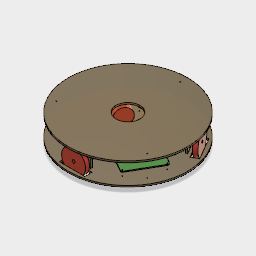
prototype (Autodesk Fusion 360 design; units mm, degrees)
Autodesk Fusion 360 part; units mm, degrees
note: some values were not read from the file. Chosen so that the rebuilt part matches the saved one: which face or edge a step refers to. Set by a fixed rule: which sketch regions a step uses.
cylinder "CylinderPrimitive1" add diameter 33 height 29 placed x (1, 0, 0) y (0, 1, 0) z (0, 0, 1) at (0, 0, 0) makes body 1 in component "motor"
cylinder "CylinderPrimitive2" add diameter 37 height 24 placed x (1, 0, 0) y (0, 1, 0) z (0, 0, 1) at (0, 0, 29) bodies 1 in component "motor"
sketch "Sketch3" plane through (0, 0, 53) normal (0, 0, 1) x (1, 0, 0) in component "motor"
  circle A0 centre (0, 0) radius 18.5
  line L0 (0, 0) -> (0, 7)
  circle A1 centre (0, 7) radius 6
  circle A2 centre (0, 0) radius 15.5
  circle A3 centre (-15.5, 0) radius 1.5
  circle A4 centre (-7.75, -13.4234) radius 1.5
  circle A5 centre (7.75, -13.4234) radius 1.5
  circle A6 centre (15.5, 0) radius 1.5
  circle A7 centre (7.75, 13.4234) radius 1.5
  circle A8 centre (-7.75, 13.4234) radius 1.5
  dimension "d7" = 7
  dimension "d8" = 12
  dimension "d13" = 31
  dimension "d14" = 3
  dimension "d20" = 360
  measures "d7" distance of A0.centre L0.end
  measures "d8" diameter of A1
  measures "d13" diameter of A2
  measures "d14" diameter of A3
cylinder "CylinderPrimitive3" add diameter 12 height 6 placed x (1, 0, 0) y (0, 1, 0) z (0, 0, 1) at (0, 7, 53) bodies 1 in component "motor"
cylinder "CylinderPrimitive4" add diameter 6 height 21 placed x (1, 0, 0) y (0, 1, 0) z (0, 0, 1) at (0, 7, 53) bodies 1 in component "motor"
extrude "Extrude2" cut sketch "Sketch3" against normal blind 10 contours A2 A6 | A2 A6 | A2 A7 | A2 A7 | A2 A5 | A2 A5 | A2 A8 | A2 A8 | A2 A4 | A2 A4 | A2 A3 | A2 A3 bodies 1 in component "motor"
move_face "OffsetFaces1" offset 15 1 faces at (4.8173, 3.9832, 0) on bodies 1 in component "motor"
sketch "Sketch7" plane through (0, 0, 29) normal (0, 0, -1) x (-1, 0, 0) in component "motor"
  circle A0 centre (0, 0) radius 18.5
  circle A1 centre (0, 0) radius 16.5
sketch "Sketch6" plane through (0, 0, 0) normal (0, 1, 0) x (1, 0, 0)
  line L0 (306.1493, 283.3069) -> (269.5493, 283.3069)
  line L1 (266.3493, 280.1069) -> (266.3493, 211.5069)
  line L2 (309.3493, 211.5069) -> (309.3493, 280.1069)
  line L3 (306.1493, 208.3069) -> (306.1493, 208.3069)
  arc A0 (306.1493, 208.3069) -> (309.3493, 211.5069) centre (306.1493, 211.5069) ccw
  arc A1 (266.3493, 211.5069) -> (269.5493, 208.3069) centre (269.5493, 211.5069) ccw
  arc A2 (309.3493, 280.1069) -> (306.1493, 283.3069) centre (306.1493, 280.1069) ccw
  arc A3 (269.5493, 283.3069) -> (266.3493, 280.1069) centre (269.5493, 280.1069) ccw
  line L4 (306.1493, 208.3069) -> (269.5493, 208.3069)
  line L5 (155.099, 257.3507) -> (209.099, 257.3507)
  line L6 (209.099, 257.3507) -> (209.099, 155.3507)
  line L7 (209.099, 155.3507) -> (155.099, 155.3507)
  line L8 (155.099, 155.3507) -> (155.099, 257.3507)
  circle A4 centre (269.5493, 211.5069) radius 1
  circle A5 centre (306.1493, 211.5069) radius 1
  circle A6 centre (269.5493, 280.1069) radius 1
  circle A7 centre (306.1493, 280.1069) radius 1
  dimension "d71" = 3.2
  dimension "d72" = 3.2
  dimension "d74" = 3.2
  dimension "d81" = 54
  dimension "d82" = 102
  dimension "d132" = 2
  dimension "d133" = 2
  dimension "d134" = 2
  dimension "d135" = 2
  measures "d71" radius of A0
  measures "d72" radius of A1
  measures "d74" radius of A3
  measures "d81" distance of L5.start L5.end
  measures "d82" distance of L5.start L7.end
  measures "d132" diameter of A4
  measures "d133" diameter of A5
  measures "d134" diameter of A6
  measures "d135" diameter of A7
move_body "Move6" bodies 1 to x (-1, 0, 0) y (0, -1, 0) z (0, 0, 1) at (0, 0, 0) in component "motor"
cylinder "CylinderPrimitive5" add diameter 60 height -11 placed x (1, 0, 0) y (0, 1, 0) z (0, 0, 1) at (0, -7, 74) separate body makes body 2 in component "motor"
sketch "Sketch10" plane through (0, 0, 0) normal (1, 0, 0) x (0, 0, -1)
  line L0 (40, 0) -> (40, 40)
other "C-Pattern5"
cylinder "CylinderPrimitive6" add diameter 50 height -8.5 placed x (1, 0, 0) y (0, 1, 0) z (0, 0, 1) at (0, -7, 74) separate body makes body 3 in component "motor"
move_body "Move7" bodies 2 to x (1, 0, 0) y (0, 1, 0) z (0, 0, 1) at (0, 0, 2) in component "motor"
move_face "OffsetFaces2" offset 2 1 faces at (7.6631, 4.2397, 65) on bodies 2 in component "motor"
sketch "Sketch12" plane through (0, -22.6, 0) normal (0, 1, 0) x (-1, 0, 0)
  line L0 (25.625, 76) -> (25.625, 63)
  line L1 (25.625, 63) -> (-25.625, 63)
  line L2 (-25.625, 63) -> (-25.625, 76)
  line L3 (-25.625, 76) -> (25.625, 76)
  circle A0 centre (0, -40) radius 125
  line L4 (25.625, 63) -> (-25.625, 63)
  line L5 (-25.625, 63) -> (-25.625, 76)
  line L6 (-25.625, 76) -> (25.625, 76)
  line L7 (25.625, 76) -> (25.625, 63)
  line L8 (-26.625, 77) -> (26.625, 77)
  line L9 (26.625, 77) -> (26.625, 62)
  line L10 (26.625, 62) -> (-26.625, 62)
  line L11 (-26.625, 62) -> (-26.625, 77)
  line L12 (-88.0125, -121.5579) -> (-114.6375, -75.4421)
  line L13 (-114.6375, -75.4421) -> (-101.6471, -67.9421)
  line L14 (-101.6471, -67.9421) -> (-75.0221, -114.0579)
  line L15 (-75.0221, -114.0579) -> (-88.0125, -121.5579)
  line L16 (114.6375, -75.4421) -> (88.0125, -121.5579)
  line L17 (88.0125, -121.5579) -> (75.0221, -114.0579)
  line L18 (75.0221, -114.0579) -> (101.6471, -67.9421)
  line L19 (101.6471, -67.9421) -> (114.6375, -75.4421)
  dimension "d127" = 1
  dimension "d129" = 360
extrude "Extrude1" add sketch "Sketch12" along normal blind 3.4 separate body contours A0 makes body 4 in component "base"
extrude "Extrude1'" add sketch "Sketch6" along normal blind 2 separate body contours L0 L1 L2 A0 A1 A2 A3 L4 makes body 5 in component "motordriver"
move_body "Move1" bodies 5 to x (0, 0, 1) y (0, 1, 0) z (-1, 0, 0) at (-246.0336, 0, -405.0116) in component "motordriver"
sketch "Sketch13" plane through (0, 0, 53) normal (0, 0, 1) x (1, 0, 0)
  line L0 (125, -19.2) -> (-125, -19.2)
  line L1 (0, 24) -> (0, -19.2) construction
  line L2 (125, -22.6) -> (-125, -22.6)
  circle A0 centre (-7.75, 13.4234) radius 1
  circle A1 centre (0, 0) radius 16.5
  circle A2 centre (0, 0) radius 16.5
  circle A3 centre (7.75, 13.4234) radius 1
  circle A4 centre (15.5, 0) radius 1
  circle A5 centre (7.75, -13.4234) radius 1
  circle A6 centre (-7.75, -13.4234) radius 1
  circle A7 centre (-15.5, 0) radius 1
  circle A8 centre (0, 0) radius 18.5
  line L3 (-18.5, 0) -> (-18.5, -22.6)
  line L4 (18.4998, 0.0775) -> (18.5948, -22.6)
  arc A9 (18.4998, 0.0775) -> (-18.5, 0) centre (0, 0) ccw
  line L5 (-18.5, -22.6) -> (18.5948, -22.6)
  circle A10 centre (0, -7) radius 6.5
  point P0 (-7.75, 13.4234)
  point P1 (7.75, 13.4234)
  point P2 (15.5, 0)
  point P3 (16.5, 0)
  point P4 (7.75, -13.4234)
  point P5 (-7.75, -13.4234)
  point P6 (-15.5, 0)
  dimension "d140" = 13
  measures "d140" diameter of A10
extrude "Extrude1''" add sketch "Sketch13" along normal blind 3.4 separate body contours L0 L2 L3 L4 L5 | L0 A8 L3 L4 | A8 L4 A9 | A1 A2 makes body 6 in component "motorHolder"
other "C-Pattern6"
combine "Combine1" operation cut target body 4 tool bodies 6 body 6 seen with x (-0.5, 0, -0.866025) y (0, 1, 0) z (0.866025, 0, -0.5) at (34.641, 0, -60) keep tools in component "base"
combine "Combine2" operation cut target body 4 tool bodies 6 keep tools in component "base"
combine "Combine3" operation cut target body 4 tool bodies 6 body 6 seen with x (-0.5, 0, 0.866025) y (0, 1, 0) z (-0.866025, 0, -0.5) at (-34.641, 0, -60) keep tools in component "base"
other "C-Pattern7"
sketch "Sketch14" plane through (0, -8, 0) normal (0, 1, 0) x (-1, 0, 0)
  circle A0 centre (-33.9396, 18.9394) radius 1
  circle A1 centre (-99.9361, -22.1699) radius 1
  circle A2 centre (-68.2396, -40.4699) radius 1
  circle A3 centre (-65.6361, 37.2394) radius 1
  line L0 (0, -40) -> (-1.5, -40)
  circle A4 centre (34.5267, -135.4623) radius 1
  circle A5 centre (-34.0733, -98.8623) radius 1
  circle A6 centre (-34.0733, -135.4623) radius 1
  circle A7 centre (34.5267, -98.8623) radius 1
  circle A8 centre (65.4094, 37.6322) radius 1
  circle A9 centre (68.0129, -40.0772) radius 1
  circle A10 centre (99.7094, -21.7772) radius 1
  circle A11 centre (33.7129, 19.3322) radius 1
  circle A12 centre (0, -40) radius 125
  circle A13 centre (0, -40) radius 125
  circle A14 centre (0, -40) radius 25
  dimension "d149" = 360
  dimension "d152" = 50
  measures "d152" diameter of A14
extrude "Extrude2'" cut sketch "Sketch14" against normal blind 85 contours A0 | A1 | A2 | A3 | A4 | A5 | A6 | A7 | A8 | A9 | A10 | A11 bodies 4 in component "base"
sketch "Sketch15" plane through (0, -8, 0) normal (0, 1, 0) x (-1, 0, 0)
  circle A0 centre (0, -40) radius 125
  circle A1 centre (0, -40) radius 125
  circle A2 centre (0, -40) radius 25
  circle A3 centre (0.2267, -149.6915) radius 1
  circle A4 centre (94.8822, 15.0421) radius 1
  circle A5 centre (-95.109, 14.6494) radius 1
  point P0 (94.8822, 15.0421)
  point P1 (-95.109, 14.6494)
  dimension "d153" = 50
  dimension "d156" = 2
  dimension "d158" = 360
  dimension "d159" = 2
  dimension "d160" = 2
  measures "d153" diameter of A2
  measures "d156" diameter of A3
  measures "d159" diameter of A4
  measures "d160" diameter of A5
extrude "Extrude3" cut sketch "Sketch15" along normal blind 80 and the other way blind 110 contours A3 | A4 | A5 bodies 4 in component "base"
extrude "Extrude1'''" add sketch "Sketch15" along normal blind 3.4 separate body makes body 7 in component "Component"
sketch "top.dfx" plane through (0, 25.4, 0) normal (0, 1, 0) x (-1, 0, 0)
  circle A0 centre (94.8822, 15.0421) radius 1
  circle A1 centre (0, -40) radius 25
  circle A2 centre (0.2267, -149.6915) radius 1
  circle A3 centre (-95.109, 14.6494) radius 1
  circle A4 centre (0, -40) radius 125
sketch "bottom.dfx" plane through (0, -19.2, 0) normal (0, 1, 0) x (-1, 0, 0)
  circle A0 centre (-95.109, 14.6494) radius 1
  circle A1 centre (0.2267, -149.6915) radius 1
  circle A2 centre (94.8822, 15.0421) radius 1
  circle A3 centre (-68.2396, -40.4699) radius 1
  circle A4 centre (34.5267, -98.8623) radius 1
  circle A5 centre (-34.0733, -135.4623) radius 1
  circle A6 centre (-65.6361, 37.2394) radius 1
  circle A7 centre (34.5267, -135.4623) radius 1
  circle A8 centre (-99.9361, -22.1699) radius 1
  circle A9 centre (68.0129, -40.0772) radius 1
  circle A10 centre (-33.9396, 18.9394) radius 1
  circle A11 centre (-34.0733, -98.8623) radius 1
  circle A12 centre (99.7094, -21.7772) radius 1
  circle A13 centre (65.4094, 37.6322) radius 1
  circle A14 centre (33.7129, 19.3322) radius 1
  line L0 (74.2348, -104.2215) -> (71.2904, -102.5215)
  line L1 (71.2904, -102.5215) -> (89.8306, -70.4088)
  line L2 (89.8306, -70.4088) -> (92.7751, -72.1088)
  line L3 (92.7751, -72.1088) -> (74.2348, -104.2215)
  line L4 (18.5, 56.4) -> (18.5, 53)
  line L5 (18.5, 53) -> (-18.5805, 53)
  line L6 (-18.5805, 53) -> (-18.5805, 56.4)
  line L7 (-18.5805, 56.4) -> (18.5, 56.4)
  line L8 (-92.7348, -72.1785) -> (-89.7904, -70.4785)
  line L9 (-89.7904, -70.4785) -> (-71.2501, -102.5912)
  line L10 (-71.2501, -102.5912) -> (-74.1946, -104.2912)
  line L11 (-74.1946, -104.2912) -> (-92.7348, -72.1785)
  line L12 (75.0221, -114.0579) -> (101.6471, -67.9421)
  line L13 (101.6471, -67.9421) -> (114.6375, -75.4421)
  line L14 (114.6375, -75.4421) -> (88.0125, -121.5579)
  line L15 (88.0125, -121.5579) -> (75.0221, -114.0579)
  line L16 (26.625, 62) -> (-26.625, 62)
  line L17 (-26.625, 62) -> (-26.625, 77)
  line L18 (-26.625, 77) -> (26.625, 77)
  line L19 (26.625, 77) -> (26.625, 62)
  line L20 (-101.6471, -67.9421) -> (-75.0221, -114.0579)
  line L21 (-75.0221, -114.0579) -> (-88.0125, -121.5579)
  line L22 (-88.0125, -121.5579) -> (-114.6375, -75.4421)
  line L23 (-114.6375, -75.4421) -> (-101.6471, -67.9421)
  circle A15 centre (0, -40) radius 125
sketch "sidePanel.dfx" plane through (0, 0, 56.4) normal (0, 0, 1) x (1, 0, 0)
  circle A0 centre (7.75, -13.4234) radius 1
  circle A1 centre (7.75, 13.4234) radius 1
  circle A2 centre (15.5, 0) radius 1
  circle A3 centre (-15.5, 0) radius 1
  circle A4 centre (-7.75, 13.4234) radius 1
  circle A5 centre (-7.75, -13.4234) radius 1
  circle A6 centre (0, -7) radius 6.5
  arc A7 (18.4998, 0.0775) -> (-18.5, 0) centre (0, 0) ccw
  line L0 (-18.5, 0) -> (-18.5, -22.6)
  line L1 (-18.5, -22.6) -> (18.5948, -22.6)
  line L2 (18.5948, -22.6) -> (18.4998, 0.0775)
component "motor" placed x (1, 0, 0) y (0, 1, 0) z (0, 0, 1) at (0, 0, 0)
component "motor" placed x (-0.5, 0, -0.866025) y (0, 1, 0) z (0.866025, 0, -0.5) at (34.641, 0, -60)
component "motor" placed x (-0.5, 0, 0.866025) y (0, 1, 0) z (-0.866025, 0, -0.5) at (-34.641, 0, -60)
component "base" placed x (1, 0, 0) y (0, 1, 0) z (0, 0, 1) at (0, 0, 0)
component "motordriver" placed x (1, 0, 0) y (0, 1, 0) z (0, 0, 1) at (0, -10, 0)
component "motorHolder" placed x (1, 0, 0) y (0, 1, 0) z (0, 0, 1) at (0, 0, 0)
component "motorHolder" placed x (-0.5, 0, -0.866025) y (0, 1, 0) z (0.866025, 0, -0.5) at (34.641, 0, -60)
component "motorHolder" placed x (-0.5, 0, 0.866025) y (0, 1, 0) z (-0.866025, 0, -0.5) at (-34.641, 0, -60)
component "motordriver" placed x (-0.5, 0, -0.866025) y (0, 1, 0) z (0.866025, 0, -0.5) at (34.641, -10, -60)
component "motordriver" placed x (-0.5, 0, 0.866025) y (0, 1, 0) z (-0.866025, 0, -0.5) at (-34.641, -10, -60)
component "Component" placed x (1, 0, 0) y (0, 1, 0) z (0, 0, 1) at (0, 30, 0)
hidden bodies 2
equation "Thickness = 3.4 mm"
equation "d130 = Thickness"
equation "d141 = Thickness"
equation "d165 = Thickness"
